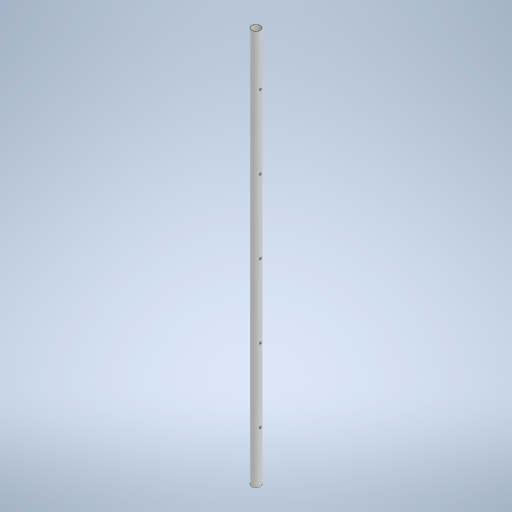
# Autodesk Inventor part: tube
Saved by Autodesk Inventor 2024 (Build 280153000, 153)
## iProperties
Created: 2023-10-26
Part Number: tube
Material: Generic
Document SubType Name: Modeling
Designer: schanen
Density: 1 g/cm^3
Appearance: Default
Author: schanen
Autodesk Inventor part; units mm, degrees
ref_plane "XZ Plane" through (0, 0, 0) normal (0, 1, 0) x (-1, 0, 0)
ref_plane "XY Plane" through (0, 0, 0) normal (0, 0, 1) x (1, 0, 0)
sketch "Sketch1" plane through (0, 0, 0) normal (0, 1, 0) x (-1, 0, 0)
  circle A0 centre (0, 0) radius 6
  circle A1 centre (0, 0) radius 5.75
  dimension "d0" = 12
  dimension "d1" = 0.25
  constraints: 2 centre point, 2 coincident
  measures "d0" diameter of A0
  measures "d1" radial gap between concentric circles of A0 A1
extrude "Extrusion1" add sketch "Sketch1" along normal blind 540
ref_plane "Work Plane1" through (6, 0, 0) normal (1, 0, 0) x (0, 1, 0)
sketch "Sketch2" plane through (6, 0, 0) normal (1, 0, 0) x (0, 1, 0)
  line L0 (0, -6) -> (0, 6) projected
  line L1 (540, -6) -> (540, 6) projected
  point P0 (0, 0)
  point P1 (270, 0)
  point P2 (0, 0)
  dimension "d5" = 540
  dimension "d6" = 270
  constraints: 1 horizontal alignment, 1 midpoint
  measures "d5" distance between parallel lines of L0 L1
  measures "d6" distance of point (0, 0) point (270, 0)
hole "Hole1" at (6, 270, 0) direction (-1, 0, 0) diameter 3 end through all
pattern_linear "Rectangular Pattern1" count 5 spacing 100 along (0, 1, 0) of "Hole1" first direction both ways yes
equation "\"d6\" = 0.5 * d5"
body "Solid1"
